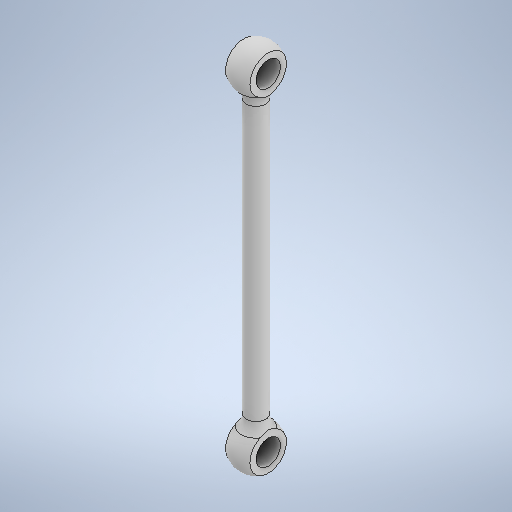
# Autodesk Inventor part: 2081
Saved by Autodesk Inventor 2025.1 (Build 291241000, 241)
## iProperties
Created: 2024-06-10
Part Number: 2081
Material: Generisch
Document SubType Name: Modeling
Designer: ffogue
Density: 1 g/cm^3
Appearance: Vorgabe
Author: ffogue
Autodesk Inventor part; units mm, degrees
ref_plane "YZ Plane" through (0, 0, 0) normal (1, 0, 0) x (0, 1, 0)
sketch "Skizze1" plane through (0, 0, 0) normal (0, 1, 0) x (-1, 0, 0)
  line L0 (0, -58) -> (0, 0)
  arc A0 (0, -62.5) -> (3, -54.6459) centre (0, -58) ccw
  line L1 (2, 0) -> (2, -52.4098)
  arc A1 (2, -52.4098) -> (3, -54.6459) centre (5, -52.4098) ccw
  line L2 (2, 0) -> (0, 0)
  line L3 (0, -62.5) -> (0, -58)
  dimension "d0" = 4.5
  dimension "d1" = 4
  dimension "d2" = 58
  dimension "d3" = 3
  constraints: 8 end point, 4 point on circle, 2 centre point, 2 tangent, 1 coincident, 1 collinear, 1 parallel, 1 perpendicular, 1 vertical alignment
  measures "d0" radius of A0
  measures "d1" diameter of L1 L0
  measures "d2" distance of L0.start L0.end
  measures "d3" radius of A1
revolve "Umdrehung1" add sketch "Skizze1" angle 360 about axis through (0, 0, -58) along (0, 0, 1)
ref_plane "Arbeitsebene1" through (0, 0, -62.5) normal (0, 0, -1) x (-1, 0, 0)
sketch "Skizze2" plane through (0, 0, -62.5) normal (0, 0, -1) x (-1, 0, 0)
  circle A0 centre (0, 0) radius 4.5 projected
  line L0 (2.5, 3.7417) -> (2.5, -3.7417)
  line L1 (-2.5, -3.7417) -> (-2.5, 3.7417)
  line L2 (0, 0) -> (0, 8.7477) construction
  line L3 (-4.5, 0) -> (4.5, 0) construction
  dimension "d6" = 5
  constraints: 8 end point, 6 point on circle, 1 horizontal, 1 parallel, 1 vertical, 1 other
  measures "d6" distance between parallel lines of L0 L1
extrude "Extrusion1" cut sketch "Skizze2" against normal blind 9 contours A0 L0 | L1 A0
sketch "Skizze3" plane through (-2.5, 0, -58) normal (-1, 0, 0) x (0, 0, 1)
  arc A0 (3.3541, 1.6583) -> (3.3541, -1.6583) centre (0, 0) ccw projected
  point P0 (58, 0)
  point P1 (0.5, 3.7081)
  point P2 (0.5, -3.7081)
  constraints: 1 coincident
hole "Bohrung1" at (-2.5, 0, -58) direction (1, 0, 0) diameter 5 end through all
ref_plane "Arbeitsebene2" through (0, 0, -24.5) normal (0, 0, 1) x (1, 0, 0)
mirror "Spiegeln1" about plane through (0, 0, -24.5) normal (0, 0, 1) of "Umdrehung1", "Extrusion1", "Bohrung1"
